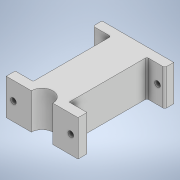
# Autodesk Inventor part: подставка лазеру
Saved by Autodesk Inventor 2022 (Build 260153000, 153)
## iProperties
Created: 2022-06-16
Part Number: подставка лазеру
Material: Типовые
Document SubType Name: Modeling
Designer: Администратор
Density: 1 g/cm^3
Appearance: По умолчанию
Author: Администратор
Autodesk Inventor part; units mm, degrees
ref_plane "YZ Plane" through (0, 0, 0) normal (1, 0, 0) x (0, 1, 0)
ref_plane "XZ Plane" through (0, 0, 0) normal (0, 1, 0) x (-1, 0, 0)
ref_plane "XY Plane" through (0, 0, 0) normal (0, 0, 1) x (1, 0, 0)
sketch "Эскиз1" plane through (0, 0, 0) normal (0, 0, 1) x (1, 0, 0)
  line L0 (-20, -10) -> (20, -10)
  line L1 (20, -10) -> (20, 10)
  line L2 (20, 10) -> (-20, 10)
  line L3 (-20, 10) -> (-20, -10)
  line L4 (-20, -10) -> (20, 10) construction
  line L5 (20, -10) -> (-20, 10) construction
  line L6 (-10, -10) -> (10, -10)
  line L7 (10, -10) -> (10, 10)
  line L8 (10, 10) -> (-10, 10)
  line L9 (-10, 10) -> (-10, -10)
  line L10 (-10, -10) -> (10, 10) construction
  line L11 (10, -10) -> (-10, 10) construction
  point P0 (0, 0)
  dimension "d0" = 40
  dimension "d1" = 20
  dimension "d2" = 20
  dimension "d3" = 20
  constraints: 24 end point, 4 midpoint, 4 parallel, 2 horizontal, 2 perpendicular
  measures "d0" distance of L2.end L1.end
  measures "d1" distance of L1.end L0.end
  measures "d2" distance of L8.end L7.end
  measures "d3" distance of L7.end L6.end
extrude "Выдавливание1" add sketch "Эскиз1" along normal blind 5 contours L3 L2 L9 L0 | L7 L2 L1 L0
extrude "Выдавливание2" add sketch "Эскиз1" along normal blind 53.359 contours L9 L2 L7 L0
fillet "Сопряжение1" radius 1 2 edges at (-10, 0, 5) (10, 0, 5)
fillet "Сопряжение2" radius 1 2 edges at (20, 0, 5) (-20, 0, 5)
sketch "Эскиз2" plane through (-20, -10, 0) normal (0, -1, 0) x (1, 0, 0)
  line L0 (30, 53.359) -> (10, 53.359) projected
  circle A0 centre (20, 53.359) radius 6
  point P0 (20, 0)
  dimension "d8" = 12
  constraints: 1 centre point, 1 midpoint
  measures "d8" diameter of A0
extrude "Выдавливание3" cut sketch "Эскиз2" against normal through all
sketch "Эскиз4" plane through (0, 0, 53.359) normal (0, 0, 1) x (1, 0, 0)
  line L0 (-20, -10) -> (20, -10) projected
  line L1 (20, 10) -> (-20, 10)
  line L2 (-20, 10) -> (-20, -10)
  line L3 (-20, -10) -> (20, -10)
  line L4 (20, -10) -> (20, 10)
  line L5 (20, 10) -> (-20, -10) construction
  line L6 (-20, 10) -> (20, -10) construction
  line L7 (6, 10) -> (6, -10) projected
  line L8 (-6, -10) -> (-6, 10) projected
  point P0 (0, 0)
  constraints: 12 end point, 2 midpoint, 2 parallel, 1 horizontal, 1 perpendicular
extrude "Выдавливание5" add sketch "Эскиз4" against normal blind 5 contours L2 L1 L8 L0 | L7 L1 L4 L0
sketch "Эскиз3" plane through (0, 0, 5) normal (0, 0, 1) x (1, 0, 0)
  circle A0 centre (16, 0) radius 1.6
  circle A1 centre (-16, 0) radius 1.6
  line L0 (20, -10) -> (20, 10) projected
  line L1 (-20, 10) -> (-20, -10) projected
  point P0 (0, 0)
  dimension "d12" = 3.2
  dimension "d13" = 3.2
  dimension "d14" = 4
  dimension "d15" = 4
  constraints: 2 centre point, 2 horizontal alignment
  measures "d12" diameter of A0
  measures "d13" diameter of A1
  measures "d14" distance from line of L0 A0.centre
  measures "d15" distance from line of L1 A1.centre
extrude "Выдавливание4" cut sketch "Эскиз3" along normal through all both and the other way through all
sketch "Эскиз5" plane through (0, 0, 53.359) normal (0, 0, 1) x (1, 0, 0)
  line L0 (-20, 10) -> (-20, -10) projected
  line L1 (20, 10) -> (-20, 10)
  line L2 (-20, 10) -> (-20, -10)
  line L3 (-20, -10) -> (20, -10)
  line L4 (20, -10) -> (20, 10)
  line L5 (20, 10) -> (-20, -10) construction
  line L6 (-20, 10) -> (20, -10) construction
  circle A0 centre (16, 0) radius 1.6 projected
  circle A1 centre (-16, 0) radius 1.6 projected
  point P0 (0, 0)
  constraints: 12 end point, 2 midpoint, 2 parallel, 1 horizontal, 1 perpendicular
extrude "Выдавливание6" add sketch "Эскиз5" along normal blind 10 separate body
extrude "Выдавливание7" cut sketch "Эскиз2" against normal through all bodies 2
sketch "Эскиз6" plane through (-20, -10, 63.359) normal (0, -1, 0) x (1, 0, 0)
  circle A0 centre (20, -10) radius 10
  line L0 (0, 0) -> (40, 0) projected
  arc A1 (26, -10) -> (14, -10) centre (20, -10) ccw projected
  line L1 (0, -10) -> (0, 0) projected
  line L2 (0, -5) -> (11.3397, -5)
  line L3 (28.6603, -5) -> (40, -5)
  line L4 (40, -10) -> (40, 0) projected
  point P0 (20, -63.359)
  point P1 (20, 0)
  constraints: 4 end point, 2 midpoint, 2 point on circle, 1 centre point, 1 concentric, 1 perpendicular, 1 point on line, 1 tangent
extrude "Выдавливание8" cut sketch "Эскиз6" against normal through all contours A0 L0 L4 L3 | L2 L1 L0 A0 bodies 2
sketch "Эскиз7" plane through (0, 0, 48.359) normal (0, 0, -1) x (-1, 0, 0)
  circle A0 centre (-16, 0) radius 1.6 projected
  line L0 (-17.5877, 2.75) -> (-14.4123, 2.75)
  line L1 (-14.4123, 2.75) -> (-12.8246, 0)
  line L2 (-12.8246, 0) -> (-14.4123, -2.75)
  line L3 (-14.4123, -2.75) -> (-17.5877, -2.75)
  line L4 (-17.5877, -2.75) -> (-19.1754, 0)
  line L5 (-19.1754, 0) -> (-17.5877, 2.75)
  circle A1 centre (16, 0) radius 1.6 projected
  line L6 (14.4123, 2.75) -> (17.5877, 2.75)
  line L7 (17.5877, 2.75) -> (19.1754, 0)
  line L8 (19.1754, 0) -> (17.5877, -2.75)
  line L9 (17.5877, -2.75) -> (14.4123, -2.75)
  line L10 (14.4123, -2.75) -> (12.8246, 0)
  line L11 (12.8246, 0) -> (14.4123, 2.75)
  point P0 (0, 0)
  dimension "d27" = 5.5
  dimension "d28" = 5.5
  constraints: 24 end point, 2 coincident, 2 vertical alignment, 26 other
  measures "d27" distance between parallel lines of L3 L0
  measures "d28" distance between parallel lines of L9 L6
extrude "Выдавливание9" cut sketch "Эскиз7" against normal blind 1 contours A0 | L0 L1 L2 L3 L4 L5 | A1 | L6 L7 L8 L9 L10 L11 bodies 1
